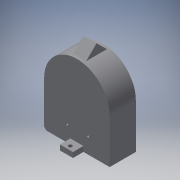
# Autodesk Inventor part: Tail3
Saved by Autodesk Inventor 2016 (Build 200138000, 138)
## iProperties
Created: 2017-03-09
Part Number: Tail3
Material: Generic
Document SubType Name: Modeling
Designer: Owner
Density: 1 g/cm^3
Appearance: Default
Author: Owner
Autodesk Inventor part; units mm, degrees
ref_plane "YZ Plane" through (0, 0, 0) normal (1, 0, 0) x (0, 1, 0)
ref_plane "XZ Plane" through (0, 0, 0) normal (0, 1, 0) x (-1, 0, 0)
sketch "Sketch1" plane through (0, 0, 0) normal (0, 0, 1) x (1, 0, 0)
  line L0 (6.1806, -38.0962) -> (6.1806, -43.1) projected
  line L1 (6.1806, -43.1) -> (32.8861, -43.1) projected
  line L2 (32.8861, -43.1) -> (32.8861, 0) projected
  arc A0 (32.8861, 0) -> (-33.1539, 0) centre (-0.1339, 0) ccw projected
  line L3 (-33.1539, 0) -> (-33.1539, -43.1) projected
  line L4 (-33.1539, -43.1) -> (-6.4839, -43.1) projected
  line L5 (-6.4839, -43.1) -> (-6.4839, -38.0962) projected
  line L6 (-6.4839, -38.0962) -> (6.1806, -38.0962) projected
  circle A1 centre (-0.1339, 0) radius 31.75
  line L7 (-31.8839, 0) -> (18.9313, 0)
  line L8 (22.7413, -43.1) -> (-31.8839, -43.1)
  line L9 (-31.8839, -43.1) -> (-31.8839, 0)
  line L10 (31.6161, 0) -> (-31.8839, 0)
  line L11 (-31.8839, 0) -> (-31.8839, -43.1)
  line L12 (-31.8839, -43.1) -> (31.6161, -43.1)
  line L13 (31.6161, -43.1) -> (31.6161, 0)
  point P0 (0, 0)
  dimension "d0" = 63.5
  constraints: 14 end point, 3 parallel, 2 horizontal, 2 point on circle, 1 centre point, 1 coincident, 1 perpendicular, 1 point on line
  measures "d0" diameter of A1
extrude "Extrusion1" add sketch "Sketch1" along normal blind 25.4 contours L6 L5 L4 L9 A1 L13 L1 L0 | L0 L8 L5 L6 | L10 L7 A1 | A1 L7 L10
sketch "Sketch2" plane through (0, 0, 0) normal (0, 0, -1) x (-1, 0, 0)
  line L0 (6.4974, -43.1) -> (-6.1987, -43.1) projected
  line L1 (-6.1987, -43.1) -> (-6.1987, -38.0962) projected
  line L2 (-6.1987, -38.0962) -> (6.4974, -38.0962) projected
  line L3 (6.4974, -38.0962) -> (6.4974, -43.1) projected
  line L4 (-6.1987, -38.0962) -> (6.5013, -38.0962)
  line L5 (6.5013, -38.0962) -> (6.5013, -33.0924)
  line L6 (6.5013, -33.0924) -> (-6.1987, -33.0924)
  line L7 (-6.1987, -33.0924) -> (-6.1987, -38.0962)
  point P0 (0, 0)
  dimension "d9" = 5.0038
  dimension "d25" = 12.7
  constraints: 8 end point, 2 parallel, 1 horizontal, 1 perpendicular
  measures "d9" distance of L6.end L1.end
  measures "d25" distance of L5.end L6.end
extrude "Extrusion4" add sketch "Sketch2" along normal blind 10.16 contours L2 L7 L6 L5 L4
sketch "Sketch4" plane through (-6.5013, -33.0924, 0) normal (0, 1, 0) x (1, 0, 0)
  line L0 (12.7, 10.16) -> (0, 10.16) projected
  line L1 (6.35, 10.16) -> (6.35, 6.35)
  circle A0 centre (6.35, 6.35) radius 2.25
  point P0 (6.5013, 0)
  dimension "d12" = 3.81
  dimension "d13" = 4.5
  constraints: 2 end point, 1 centre point, 1 coincident, 1 midpoint, 1 vertical
  measures "d12" distance of L1.start L1.end
  measures "d13" diameter of A0
extrude "Extrusion5" cut sketch "Sketch4" against normal blind 10.16
sketch "Sketch5" plane through (0, 0, 25.4) normal (0, 0, 1) x (1, 0, 0)
  line L0 (-4.5713, -43.1) -> (1.7787, -43.1)
  line L1 (1.7787, -43.1) -> (-10.9213, -43.1)
  line L2 (-10.9213, -43.1) -> (6.2237, -43.1)
  line L3 (6.2237, -43.1) -> (6.2237, -38.0962)
  line L4 (6.2237, -38.0962) -> (-10.9213, -38.0962)
  line L5 (-0.1339, -43.1) -> (6.2161, -43.1)
  line L6 (6.2161, -43.1) -> (-6.4839, -43.1)
  line L7 (-6.4839, -43.1) -> (6.2237, -43.1)
  line L8 (6.2237, -43.1) -> (6.2237, -38.0962)
  line L9 (6.2237, -38.0962) -> (-6.4839, -38.0962)
  line L10 (-6.4839, -38.0962) -> (-6.4839, -43.1)
  point P0 (0, 0)
  dimension "d16" = 6.35
  dimension "d17" = 12.7
  dimension "d18" = 5.0038
  dimension "d26" = 6.35
  dimension "d27" = 12.7
  dimension "d28" = 5.0038
  constraints: 22 end point, 3 parallel, 2 horizontal, 2 perpendicular, 1 point on line
  measures "d16" distance of L0.start L0.end
  measures "d17" distance of L0.end L1.end
  measures "d18" distance of L2.end L3.end
  measures "d26" distance of L5.start L5.end
  measures "d27" distance of L5.end L6.end
  measures "d28" distance of L7.end L8.end
extrude "Extrusion6" add sketch "Sketch5" along normal blind 10.16
sketch "Sketch7" plane through (-6.4839, -38.0962, 25.4) normal (0, 1, 0) x (1, 0, 0)
  line L0 (12.7076, -10.16) -> (0, -10.16) projected
  line L1 (6.3538, -10.16) -> (6.3538, -6.35)
  circle A0 centre (6.3538, -6.35) radius 1.75
  point P0 (6.4839, 25.4)
  dimension "d29" = 3.81
  dimension "d30" = 3.5
  constraints: 2 end point, 1 centre point, 1 coincident, 1 midpoint, 1 vertical
  measures "d29" distance of L1.start L1.end
  measures "d30" diameter of A0
extrude "Extrusion8" cut sketch "Sketch7" against normal blind 10.16
ref_plane "Work Plane1" through (-0.1339, -43.1, 0) normal (-1, 0, 0) x (0, 0, 1)
sketch "Sketch8" plane through (-0.1339, -43.1, 0) normal (-1, 0, 0) x (0, 0, 1)
  line L0 (0, 74.85) -> (0, 43.1) projected
  line L1 (0, 74.85) -> (2.7051, 74.85)
  line L2 (0, 74.85) -> (25.4, 74.85) projected
  line L3 (2.7051, 74.85) -> (22.6949, 74.85)
  line L4 (22.6949, 74.85) -> (12.6873, 74.85)
  line L5 (12.6873, 74.85) -> (12.6873, 84.8576)
  line L6 (12.6873, 84.8576) -> (22.6949, 74.85)
  line L7 (12.6873, 84.8576) -> (2.7051, 74.85)
  dimension "d34" = 2.7051
  dimension "d35" = 19.9898
  dimension "d36" = 10.0076
  dimension "d37" = 10.0076
  constraints: 12 end point, 3 point on line, 1 perpendicular
  measures "d34" distance of L0.start L1.end
  measures "d35" distance of L1.end L3.end
  measures "d36" distance of L3.end L4.end
  measures "d37" distance of L4.end L5.end
extrude "Extrusion9" add sketch "Sketch8" along normal mid plane 12.7
sketch "Sketch9" plane through (0, 0, 0) normal (0, 0, -1) x (-1, 0, 0)
  ellipse E0 centre (-12.3919, -27.5683) end of major axis (-12.3919, -26.3183) minor radius 1.25 projected
  ellipse E1 centre (11.7381, -27.5683) end of major axis (11.7381, -26.3183) minor radius 1.25 projected
  line L0 (-12.3919, -27.5683) -> (-10.3919, -27.5683)
  line L1 (11.7381, -27.5683) -> (9.7381, -27.5683)
  circle A0 centre (-10.3919, -27.5683) radius 1.25
  circle A1 centre (-10.3919, -27.5683) radius 1.25
  circle A2 centre (9.7381, -27.5683) radius 1.2446
  point P0 (0, 0)
  dimension "d40" = 2
  dimension "d41" = 2
  dimension "d44" = 2.4892
  constraints: 4 end point, 3 centre point, 2 coincident, 2 horizontal, 1 concentric, 2 other
  measures "d40" distance of L0.start L0.end
  measures "d41" distance of L1.start L1.end
  measures "d44" diameter of A2
extrude "Extrusion10" cut sketch "Sketch9" against normal blind 25.4 contours A0 L0 E0 | E0 A0 | E0 L0 A0 | A2 L1 E1 | E1 A2 | E1 L1 A2 picked at (-9.8215, -27.4653) picked at (9.1713, -27.6709)
body "Solid1"
